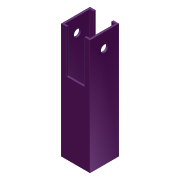
# Autodesk Inventor part: PivotLeverBar
Saved by Autodesk Inventor 2012 (Build 160160000, 160)
## iProperties
Created: 2013-01-19
Part Number: PivotLeverBar
Material: Aluminum-6061
Document SubType Name: Modeling
Designer: JesseK
Density: 2.71 g/cm^3
Mass: 66.7623 g
Surface Area: 166.935 cm^2
Volume: 24.6355 cm^3
Author: JesseK
Autodesk Inventor part; units mm, degrees
ref_plane "YZ Plane" through (0, 0, 0) normal (1, 0, 0) x (0, 1, 0)
ref_plane "XZ Plane" through (0, 0, 0) normal (0, 1, 0) x (-1, 0, 0)
ref_plane "XY Plane" through (0, 0, 0) normal (0, 0, 1) x (1, 0, 0)
sketch "Sketch1" plane through (0, 0, 0) normal (0, 0, 1) x (1, 0, 0)
  line L0 (0, 0) -> (25.4, 0)
  line L1 (25.4, 0) -> (25.4, 101.6)
  line L2 (25.4, 101.6) -> (0, 101.6)
  line L3 (0, 101.6) -> (0, 0)
  dimension "d0" = 25.4
  dimension "d1" = 101.6
  constraints: 8 end point, 2 parallel, 1 horizontal, 1 perpendicular
  measures "d0" distance between parallel lines of L1 L3
  measures "d1" distance of L2.end L0.start
extrude "Extrusion1" add sketch "Sketch1" along normal blind 25.4
shell "Shell1" thickness 3.175 removed faces 2 at (16.9333, 101.6, 16.9333) at (8.4667, 0, 8.4667)
sketch "Sketch2" plane through (25.4, 0, 0) normal (1, 0, 0) x (0, 0, -1)
  line L0 (0, 0) -> (0, 101.6) projected
  circle A0 centre (-12.7, 88.9) radius 3.175
  line L1 (0, 0) -> (-25.4, 0) projected
  dimension "d8" = 6.35
  dimension "d9" = 12.7
  dimension "d13" = 88.9
  constraints: 1 centre point
  measures "d8" diameter of A0
  measures "d9" distance from line of L0 A0.centre
  measures "d13" distance from line of L1 A0.centre
extrude "Extrusion2" cut sketch "Sketch2" against normal through all
sketch "Sketch3" plane through (0, 0, 0) normal (0, 0, -1) x (-1, 0, 0)
  line L0 (0, 101.6) -> (0, 0) projected
  line L1 (-25.4, 101.6) -> (0, 101.6) projected
  line L2 (-25.4, 0) -> (-25.4, 101.6) projected
  line L3 (-20.6375, 101.6) -> (-4.7625, 101.6)
  line L4 (-4.7625, 101.6) -> (-4.7625, 63.5)
  line L5 (-4.7625, 63.5) -> (-20.6375, 63.5)
  line L6 (-20.6375, 63.5) -> (-20.6375, 101.6)
  dimension "d14" = 38.1
  dimension "d15" = 4.7625
  dimension "d16" = 4.7625
  constraints: 8 end point, 2 parallel, 1 horizontal, 1 perpendicular, 1 point on line
  measures "d14" distance of L3.end L4.end
  measures "d15" distance between parallel lines of L0 L4
  measures "d16" distance between parallel lines of L2 L6
extrude "Extrusion3" cut sketch "Sketch3" against normal blind 25.4
body "Solid1"
